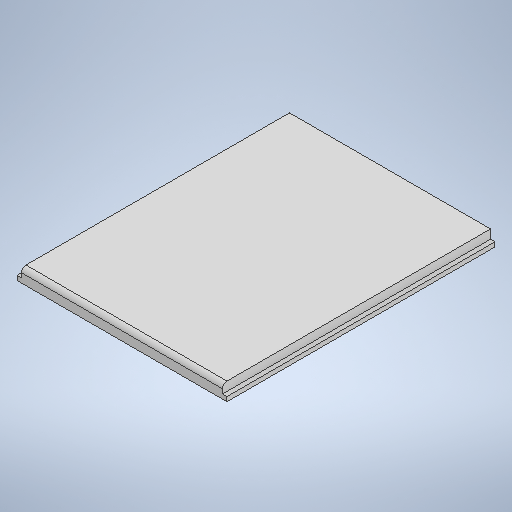
# Autodesk Inventor part: upper coverr
Saved by Autodesk Inventor 2025.4 (Build 294407000, 407)
## iProperties
Created: 2026-04-11
Part Number: upper coverr
Material: Generic
Document SubType Name: Modeling
Designer: Amir
Density: 1 g/cm^3
Appearance: Default
Author: Amir
## iProperties of the stored document upper coverr_3DPrint.ipt
Created: 2026-04-12
Part Number: upper coverr_3DPrint
Material: Generic
Document SubType Name: Modeling
Designer: Amir
Density: 1 g/cm^3
Appearance: Default
Author: Amir
Autodesk Inventor part; units mm, degrees
ref_plane "YZ Plane" through (0, 0, 0) normal (1, 0, 0) x (0, 1, 0)
ref_plane "XZ Plane" through (0, 0, 0) normal (0, 1, 0) x (-1, 0, 0)
ref_plane "XY Plane" through (0, 0, 0) normal (0, 0, 1) x (1, 0, 0)
sketch "Sketch1" plane through (0, 0, 0) normal (0, 0, 1) x (1, 0, 0)
  line L0 (-22.5075, -0.5954) -> (22.4925, -0.5954)
  line L1 (22.4925, -0.5954) -> (22.4925, 0.4046)
  line L2 (-22.5075, -0.5954) -> (-23.5075, -0.5954)
  line L3 (-23.5075, -0.5954) -> (-23.5075, 0.4046)
  line L4 (-22.5075, 2.4046) -> (22.4925, 2.4046)
  line L5 (22.4925, 2.4046) -> (22.4925, 0.4046)
  line L6 (22.4925, 0.4046) -> (23.4925, 0.4046)
  line L7 (23.4925, 0.4046) -> (23.4925, -0.5954)
  line L8 (23.4925, -0.5954) -> (22.4925, -0.5954)
  line L9 (-23.5075, 0.4046) -> (-22.5075, 0.4046)
  line L10 (-22.5075, 2.4046) -> (-22.5075, 0.4046)
  point P0 (0, 0)
  dimension "d2" = 1
  dimension "d3" = 1
  dimension "d5" = 1
  dimension "d6" = 1
  dimension "d7" = 3
  dimension "d11" = 2
  constraints: 22 end point, 5 perpendicular, 3 horizontal, 1 point on line, 1 vertical
  measures "d2" distance of L0.start L2.end
  measures "d3" distance of L2.end L3.end
  measures "d5" distance of L1.end L6.end
  measures "d6" distance of L6.end L7.end
  measures "d7" distance between parallel lines of L4 L0
  measures "d11" distance between parallel lines of L6 L4
extrude "Extrusion1" add sketch "Sketch1" along normal blind 60
fillet "Fillet1" radius 1 1 edges at (-0.0075, 2.4046, 60)
body "Solid1"
